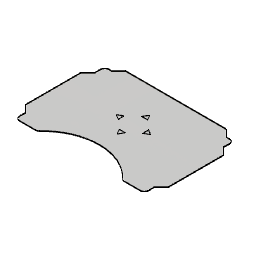
cover_window (Autodesk Fusion 360 design; units mm, degrees)
Autodesk Fusion 360 part; units mm, degrees
sketch "Esquisse1" plane through (0, 0, 0) normal (0, 1, 0) x (1, 0, 0)
  line L0 (-367.4671, -125) -> (350, -125) construction
  arc A0 (209.2489, -218.6842) -> (223.8346, -225) centre (223.8346, -205) ccw
  arc A1 (-223.8346, -225) -> (-209.2489, -218.6842) centre (-223.8346, -205) ccw
  arc A2 (209.2489, -218.6842) -> (-209.2489, -218.6842) centre (0, -415) ccw
  line L1 (-305, 225) -> (305, 225)
  line L2 (325, 205) -> (325, -205)
  line L3 (305, -225) -> (223.8346, -225)
  line L4 (-325, -205) -> (-325, 205)
  arc A3 (325, 205) -> (305, 225) centre (305, 205) ccw
  line L5 (325, 225) -> (-325, -225) construction
  arc A4 (-305, 225) -> (-325, 205) centre (-305, 205) ccw
  arc A5 (-325, -205) -> (-305, -225) centre (-305, -205) ccw
  line L6 (-305, -225) -> (-223.8346, -225)
  line L7 (-325, 225) -> (325, -225) construction
  arc A6 (305, -225) -> (325, -205) centre (305, -205) ccw
  line L8 (215, -225) -> (325, -225)
  point P0 (-215, -225)
  dimension "d12" = 650
  dimension "d13" = 450
  dimension "d14" = 110
  dimension "d15" = 110
  dimension "d16" = 100
  dimension "d20" = 190
  dimension "d21" = 20
  constraint horizontal L1
  constraint perpendicular L1 L2
  constraint parallel L1 L3
  constraint parallel L2 L4
  constraint coincident origin L7
  constraint coincident origin L5
  constraint coincident P0 L3
  constraint perpendicular L0 L2
  constraint perpendicular L2 L8
  constraint tangent A0 A2
  constraint tangent A0 L3
  constraint coincident L7.end L3
  constraint coincident L7.end L2
  constraint tangent L3 A6
  constraint tangent L2 A6
  constraint equal A0 A6
  constraint coincident L5.start L1
  constraint coincident L5.start L2
  constraint tangent L1 A3
  constraint tangent L2 A3
  constraint equal A0 A3
  constraint coincident L7.start L1
  constraint coincident L7.start L4
  constraint tangent L1 A4
  constraint tangent L4 A4
  constraint equal A0 A4
  constraint coincident L5.end L4
  constraint coincident L5.end L6
  constraint tangent L4 A5
  constraint tangent A5 L6
  constraint equal A0 A5
  constraint coincident P0 L6
  constraint coincident P0 A2
  constraint tangent A1 L6
  constraint tangent A1 A2
  constraint equal A0 A1
  measures "d12" distance of L5.start L7.start
  measures "d13" distance of L5.end L7.start
  measures "d14" distance of P0 L4
  measures "d15" distance of L8.start L2
  measures "d16" distance of L0 L3
  measures "d20" distance of A2.centre L3
  measures "d21" radius of A0
extrude "Extrusion1" add sketch "Esquisse1" along normal blind 3
sketch "Esquisse2" plane through (0, 3, 0) normal (0, 1, 0) x (-1, 0, 0)
  arc A0 (325, 205) -> (305, 225) centre (305, 205) ccw
  line L0 (305, 225) -> (223.8346, 225)
  arc A1 (223.8346, 225) -> (209.2489, 218.6842) centre (223.8346, 205) ccw
  arc A2 (-209.2489, 218.6842) -> (209.2489, 218.6842) centre (0, 415) ccw
  arc A3 (-209.2489, 218.6842) -> (-223.8346, 225) centre (-223.8346, 205) ccw
  line L1 (-223.8346, 225) -> (-305, 225)
  arc A4 (-305, 225) -> (-325, 205) centre (-305, 205) ccw
  line L2 (-325, 205) -> (-325, -205)
  arc A5 (-325, -205) -> (-305, -225) centre (-305, -205) ccw
  line L3 (-305, -225) -> (305, -225)
  arc A6 (305, -225) -> (325, -205) centre (305, -205) ccw
  line L4 (325, -205) -> (325, 205)
  line L5 (14.7224, 11.5) -> (0, 37)
  line L6 (-14.7224, 11.5) -> (14.7224, 11.5)
  line L7 (0, 37) -> (-14.7224, 11.5)
  line L8 (-61.5, -59.7224) -> (-61.5, -30.2776)
  line L9 (-87, -45) -> (-61.5, -59.7224)
  line L10 (-61.5, -30.2776) -> (-87, -45)
  line L11 (-14.7224, -101.5) -> (0, -127)
  line L12 (0, -127) -> (14.7224, -101.5)
  line L13 (14.7224, -101.5) -> (-14.7224, -101.5)
  line L14 (61.5, -30.2776) -> (61.5, -59.7224)
  line L15 (388.9907, -50) -> (-400, -50) construction
  line L16 (87, -45) -> (61.5, -30.2776)
  line L17 (61.5, -59.7224) -> (87, -45)
  point P0 (70, -45)
  point P1 (0, -110)
  point P2 (0, 20)
  dimension "d46" = 5
  dimension "d48" = 70
  dimension "d52" = 17
  measures "d46" distance of P0 L15
  measures "d48" distance of P2 L15
  measures "d52" distance of P1 L11.end
extrude "Extrusion2" cut sketch "Esquisse2" against normal blind 1 contours L5 L6 L7 | L8 L9 L10 | L11 L12 L13 | L14 L16 L17
sketch "Esquisse3" plane through (0, 3, 0) normal (0, 1, 0) x (-1, 0, 0)
  line L0 (0, -127) -> (-14.7224, -101.5)
  line L1 (-14.7224, -101.5) -> (14.7224, -101.5)
  line L2 (14.7224, -101.5) -> (0, -127)
  line L3 (-61.5, -59.7224) -> (-87, -45)
  line L4 (-87, -45) -> (-61.5, -30.2776)
  line L5 (-61.5, -30.2776) -> (-61.5, -59.7224)
  line L6 (61.5, -30.2776) -> (87, -45)
  line L7 (87, -45) -> (61.5, -59.7224)
  line L8 (61.5, -59.7224) -> (61.5, -30.2776)
  line L9 (14.7224, 11.5) -> (-14.7224, 11.5)
  line L10 (-14.7224, 11.5) -> (0, 37)
  line L11 (0, 37) -> (14.7224, 11.5)
  arc A0 (325, 205) -> (305, 225) centre (305, 205) ccw
  line L12 (305, 225) -> (223.8346, 225)
  arc A1 (223.8346, 225) -> (209.2489, 218.6842) centre (223.8346, 205) ccw
  arc A2 (-209.2489, 218.6842) -> (209.2489, 218.6842) centre (0, 415) ccw
  arc A3 (-209.2489, 218.6842) -> (-223.8346, 225) centre (-223.8346, 205) ccw
  line L13 (-223.8346, 225) -> (-305, 225)
  arc A4 (-305, 225) -> (-325, 205) centre (-305, 205) ccw
  line L14 (-325, 205) -> (-325, -205)
  arc A5 (-325, -205) -> (-305, -225) centre (-305, -205) ccw
  line L15 (-305, -225) -> (305, -225)
  arc A6 (305, -225) -> (325, -205) centre (305, -205) ccw
  line L16 (325, -205) -> (325, 205)
  line L17 (0, -325) -> (0, 225)
  line L18 (290, -225) -> (255, -260)
  line L19 (255, -260) -> (0, -260)
  line L20 (325, -175) -> (360, -140)
  line L21 (360, -140) -> (360, 140)
  line L22 (360, 140) -> (325, 175)
  line L23 (-255, -260) -> (0, -260)
  line L24 (-290, -225) -> (-255, -260)
  line L25 (-325, -175) -> (-360, -140)
  line L26 (-360, -140) -> (-360, 140)
  line L27 (-360, 140) -> (-325, 175)
  dimension "d22" = 35
  dimension "d23" = 45
  dimension "d24" = 580
  dimension "d25" = 35
  dimension "d26" = 45
  dimension "d27" = 45
  dimension "d28" = 350
  dimension "d30" = 30
  constraint vertical L17
  constraint coincident L15 L18.start
  constraint coincident L17 L19.end
  constraint perpendicular L17 L19
  constraint coincident L16 L20.start
  constraint parallel L18 L20
  constraint parallel L16 L21
  constraint coincident L16 L22.end
  constraint perpendicular L20 L22
  constraint symmetric L17 L18.start L24.start
  constraint symmetric L17 L18.end L23.start
  constraint symmetric L17 L19.end L23.end
  constraint symmetric L17 L20.start L25.start
  constraint symmetric L17 L20.end L25.end
  constraint symmetric L17 L21.end L26.end
  constraint symmetric L17 L22.end L27.end
  measures "d22" distance of L15 L19
  measures "d23" angle of L15 L18
  measures "d25" distance of L16 L21
  measures "d26" angle of L16 L20
  measures "d27" angle of L16 L22
  measures "d28" distance of L20.start L22.end
  measures "d30" distance of A6.end L20.start
extrude "Extrusion3" add sketch "Esquisse3" against normal up to surface (3 mm away) contours L15 L17 L23 L24 | L15 L17 L18 L19 | L14 L25 L26 L27 | L16 L20 L21 L22
sketch "Esquisse4" plane through (0, 3, 0) normal (0, 1, 0) x (-1, 0, 0)
  line L0 (0, -127) -> (-14.7224, -101.5)
  line L1 (-14.7224, -101.5) -> (14.7224, -101.5)
  line L2 (14.7224, -101.5) -> (0, -127)
  line L3 (-61.5, -59.7224) -> (-87, -45)
  line L4 (-87, -45) -> (-61.5, -30.2776)
  line L5 (-61.5, -30.2776) -> (-61.5, -59.7224)
  line L6 (61.5, -30.2776) -> (87, -45)
  line L7 (87, -45) -> (61.5, -59.7224)
  line L8 (61.5, -59.7224) -> (61.5, -30.2776)
  line L9 (14.7224, 11.5) -> (-14.7224, 11.5)
  line L10 (-14.7224, 11.5) -> (0, 37)
  line L11 (0, 37) -> (14.7224, 11.5)
  arc A0 (325, 205) -> (305, 225) centre (305, 205) ccw
  line L12 (305, 225) -> (223.8346, 225)
  arc A1 (223.8346, 225) -> (209.2489, 218.6842) centre (223.8346, 205) ccw
  arc A2 (-209.2489, 218.6842) -> (209.2489, 218.6842) centre (0, 415) ccw
  arc A3 (-209.2489, 218.6842) -> (-223.8346, 225) centre (-223.8346, 205) ccw
  line L13 (-223.8346, 225) -> (-305, 225)
  arc A4 (-305, 225) -> (-325, 205) centre (-305, 205) ccw
  line L14 (-325, 205) -> (-325, 175)
  line L15 (-325, 175) -> (-360, 140)
  line L16 (-360, 140) -> (-360, -140)
  line L17 (-360, -140) -> (-325, -175)
  line L18 (-325, -175) -> (-325, -205)
  arc A5 (-325, -205) -> (-305, -225) centre (-305, -205) ccw
  line L19 (-305, -225) -> (-290, -225)
  line L20 (-290, -225) -> (-255, -260)
  line L21 (-255, -260) -> (255, -260)
  line L22 (255, -260) -> (290, -225)
  line L23 (290, -225) -> (305, -225)
  arc A6 (305, -225) -> (325, -205) centre (305, -205) ccw
  line L24 (325, -205) -> (325, -175)
  line L25 (325, -175) -> (360, -140)
  line L26 (360, -140) -> (360, 140)
  line L27 (360, 140) -> (325, 175)
  line L28 (325, 175) -> (325, 205)
